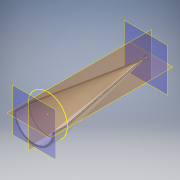
# Autodesk Inventor part: Головной обтекатель
Saved by Autodesk Inventor 2017 (Build 210142000, 142)
## iProperties
Part Number: Головной обтекатель
Material: Типовые
Document SubType Name: Modeling
Designer: Arseny Radushin
Density: 1 g/cm^3
Appearance: По умолчанию
Author: Arseny Radushin
Autodesk Inventor part; units mm, degrees
sketch "Эскиз1" plane through (0, 0, 0) normal (0, 1, 0) x (-1, 0, 0)
  circle A0 centre (0, 0) radius 15
  circle A1 centre (0, 0) radius 16
  dimension "d0" = 30
  dimension "d1" = 32
  constraints: 2 centre point, 2 coincident
  measures "d0" diameter of A0
  measures "d1" diameter of A1
extrude "Выдавливание1" add sketch "Эскиз1" along normal blind 11
ref_plane "РабПлоскость1" through (0, 91, 0) normal (0, 1, 0) x (1, 0, 0)
sketch "Эскиз3" plane through (0, 91, 0) normal (0, 1, 0) x (1, 0, 0)
  point P0 (0, 0)
  point P1 (0, 0)
  point P2 (0, 0)
  constraints: 2 coincident
sketch "Эскиз4" plane through (0, 11, 0) normal (0, 1, 0) x (1, 0, 0)
  circle A0 centre (0, 0) radius 16 projected
sketch "Эскиз6" plane through (0, 0, 0) normal (0, 0, 1) x (1, 0, 0)
  line L0 (0, 91) -> (16, 11)
  line L1 (0, 111.2721) -> (0, 58.6292)
  line L2 (16, 11) -> (0, 11)
  line L3 (16, 11) -> (-16, 11) projected
  line L4 (0, 91) -> (0, 11)
  point P0 (0, 0)
  dimension "d10" = 16
  dimension "d11" = 3.9757
  dimension "d12" = 6.3484
  constraints: 8 end point, 1 midpoint, 1 perpendicular, 1 vertical
  measures "d10" distance from line of L0.end L1
  measures "d11" distance from line of L1.start L0
  measures "d12" distance from line of L1.end L0
revolve "Вращение1" add sketch "Эскиз6" angle 360 about axis through (0, 111.2721, 0) along (0, -1, 0)
sketch "Эскиз7" plane through (0, 0, 0) normal (0, 0, 1) x (1, 0, 0)
  line L0 (15, 11) -> (0, 86)
  line L1 (0, 91) -> (16, 11) projected
  line L2 (0, 109.2) -> (0, -18.2) projected
  line L3 (0, 86) -> (0, 11)
  line L4 (-15, 11) -> (15, 11) projected
  line L5 (0, 11) -> (15, 11)
  point P0 (0, 0)
  constraints: 6 end point, 2 point on line, 1 horizontal, 1 parallel
revolve "Вращение2" cut sketch "Эскиз7" angle 360 about axis through (0, 86, 0) along (0, -1, 0)
